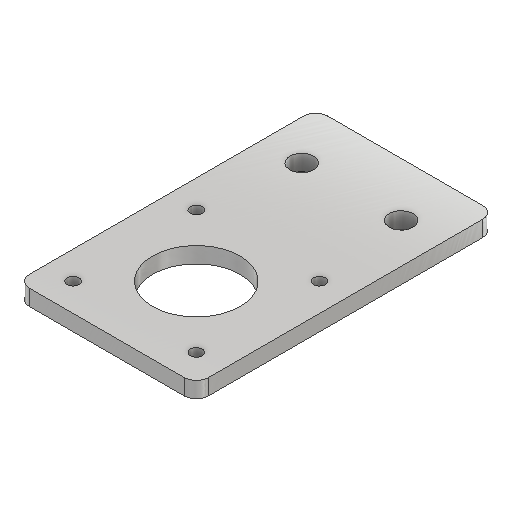
# Autodesk Inventor part: LC_ALU_4mm_Z_Axis_Stepper_Mount
Saved by Autodesk Inventor 2026.1 (Build 301233000, 233)
## iProperties
Created: 2016-06-24
Part Number: LC_ALU_4mm_Z_Axis_Stepper_Mount
Material: Ogólny
Document SubType Name: Modeling
Designer: Andrzej
Density: 1 g/cm^3
Appearance: Obrobione - aluminium
Mass: 11.4084 g
Surface Area: 71.8451 cm^2
Volume: 11.4084 cm^3
Author: Andrzej
Autodesk Inventor part; units mm, degrees
ref_plane "YZ Plane" through (0, 0, 0) normal (1, 0, 0) x (0, 1, 0)
ref_plane "XZ Plane" through (0, 0, 0) normal (0, 1, 0) x (-1, 0, 0)
ref_plane "XY Plane" through (0, 0, 0) normal (0, 0, 1) x (1, 0, 0)
sketch "Szkic1" plane through (0, 0, 0) normal (0, 0, 1) x (1, 0, 0)
  line L0 (-9.5608, 1.5423) -> (35.4392, 1.5423)
  line L1 (35.4392, 1.5423) -> (35.4392, -73.4577)
  line L2 (26.8018, -148.3336) -> (-18.1982, -148.3336)
  line L3 (-9.5608, -73.4577) -> (-9.5608, 1.5423)
  line L4 (33.9392, -71.9577) -> (-8.0608, -71.9577)
  line L5 (-8.0608, -71.9577) -> (-8.0608, -29.9577)
  line L6 (-8.0608, -29.9577) -> (33.9392, -29.9577)
  line L7 (33.9392, -29.9577) -> (33.9392, -71.9577)
  line L8 (-9.5608, -73.4577) -> (35.4392, -73.4577)
  circle A0 centre (12.9392, -50.9577) radius 11
  circle A1 centre (-2.5608, -35.4577) radius 1.5
  circle A2 centre (28.4392, -35.4577) radius 1.5
  circle A3 centre (-2.5608, -66.4577) radius 1.5
  circle A4 centre (28.4392, -66.4577) radius 1.5
  circle A5 centre (0.4392, -11.9577) radius 3
  circle A6 centre (25.4392, -11.9577) radius 3
  point P0 (0, 0)
  dimension "d0" = 45
  dimension "d1" = 75
  dimension "d2" = 42
  dimension "d3" = 42
  dimension "d4" = 5.5
  dimension "d5" = 5.5
  dimension "d6" = 5.5
  dimension "d7" = 5.5
  dimension "d8" = 5.5
  dimension "d9" = 5.5
  dimension "d10" = 5.5
  dimension "d11" = 5.5
  dimension "d12" = 21
  dimension "d13" = 21
  dimension "d24" = 45
  dimension "d25" = 1.5
  dimension "d26" = 1.5
  dimension "d27" = 13.5
  dimension "d28" = 13.5
  dimension "d29" = 22
  dimension "d30" = 3
  dimension "d31" = 3
  dimension "d32" = 3
  dimension "d33" = 3
  dimension "d43" = 10
  dimension "d44" = 10
  dimension "d45" = 6
  dimension "d46" = 6
  constraints: 18 end point, 7 centre point, 7 coincident, 4 parallel, 3 horizontal, 2 perpendicular
  measures "d0" distance of L2.start L2.end
  measures "d1" distance of L1.end L0.end
  measures "d2" distance of L5.end L7.start
  measures "d3" distance of L5.start L5.end
  measures "d4" distance from line of L7 point (28.439, -66.458)
  measures "d5" distance from line of L4 point (28.439, -66.458)
  measures "d6" distance from line of L4 point (-2.561, -66.458)
  measures "d7" distance from line of L5 point (-2.561, -66.458)
  measures "d8" distance from line of L7 point (28.439, -35.458)
  measures "d9" distance from line of L6 point (28.439, -35.458)
  measures "d10" distance from line of L6 point (-2.561, -35.458)
  measures "d11" distance from line of L5 point (-2.561, -35.458)
  measures "d12" distance from line of L4 point (12.939, -50.958)
  measures "d13" distance from line of L7 point (12.939, -50.958)
  measures "d24" distance of L3.start L1.end
  measures "d25" distance between parallel lines of L3 L5
  measures "d26" distance between parallel lines of L8 L4
  measures "d27" distance from line of L0 point (0.439, -11.958)
  measures "d28" distance from line of L0 point (25.439, -11.958)
  measures "d29" diameter of A0
  measures "d30" diameter of A1
  measures "d31" diameter of A2
  measures "d32" diameter of A3
  measures "d33" diameter of A4
  measures "d43" distance from line of L3 point (0.439, -11.958)
  measures "d44" distance from line of L1 point (25.439, -11.958)
  measures "d45" diameter of A5
  measures "d46" diameter of A6
extrude "Wyciągnięcie proste2" add sketch "Szkic1" along normal blind 4 contours L0 L1 L8 L3 | L4 L5 L6 L7
fillet "Zaokrąglenie1" radius 3 4 edges at (35.4392, -73.4577, 2) (-9.5608, -73.4577, 2) (35.4392, 1.5423, 2) (-9.5608, 1.5423, 2)
equation "\"d5\" = d4"
equation "\"d6\" = d4"
equation "\"d7\" = d4"
equation "\"d8\" = d4"
equation "\"d9\" = d4"
equation "\"d10\" = d4"
equation "\"d11\" = d4"
equation "\"d12\" = 0.5 * d3"
equation "\"d13\" = d12"
equation "\"d25\" = -0.5 * d2 + 0.5 * d24"
equation "\"d28\" = d27"
